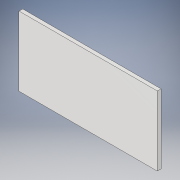
# Autodesk Inventor part: toptable
Saved by Autodesk Inventor 2017 (Build 210142000, 142)
## iProperties
Created: 2018-08-24
Part Number: toptable
Material: Generic
Document SubType Name: Modeling
Designer: emmacarlisle
Density: 1 g/cm^3
Appearance: Smooth - White
Author: emmacarlisle
Autodesk Inventor part; units mm, degrees
ref_plane "YZ Plane" through (0, 0, 0) normal (1, 0, 0) x (0, 1, 0)
ref_plane "XZ Plane" through (0, 0, 0) normal (0, 1, 0) x (-1, 0, 0)
ref_plane "XY Plane" through (0, 0, 0) normal (0, 0, 1) x (1, 0, 0)
sketch "Sketch1" plane through (0, 0, 0) normal (0, 0, 1) x (1, 0, 0)
  line L0 (0, 0) -> (1495, 0)
  line L1 (1495, 0) -> (1495, 750)
  line L2 (1495, 750) -> (0, 750)
  line L3 (0, 750) -> (0, 0)
  dimension "d0" = 1495
  dimension "d1" = 750
  constraints: 8 end point, 2 parallel, 1 horizontal, 1 perpendicular
  measures "d0" distance of L1.end L2.end
  measures "d1" distance of L0.end L1.end
extrude "Extrusion1" add sketch "Sketch1" along normal blind 40
body "Solid1"
